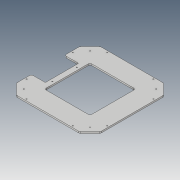
# Autodesk Inventor part: topPlate
Saved by Autodesk Inventor 2018 (Build 220112000, 112)
## iProperties
Created: 2019-11-22
Part Number: topPlate
Material: Generic
Document SubType Name: Modeling
Designer: anirudh
Density: 1 g/cm^3
Appearance: Default
Author: anirudh
Autodesk Inventor part; units mm, degrees
ref_plane "YZ Plane" through (0, 0, 0) normal (1, 0, 0) x (0, 1, 0)
ref_plane "XZ Plane" through (0, 0, 0) normal (0, 1, 0) x (-1, 0, 0)
ref_plane "XY Plane" through (0, 0, 0) normal (0, 0, 1) x (1, 0, 0)
sketch "Sketch1" plane through (0, 0, 0) normal (0, 1, 0) x (-1, 0, 0)
  line L0 (304.8, -38.1) -> (304.8, -266.7)
  line L1 (266.7, -304.8) -> (38.1, -304.8)
  line L2 (0, -266.7) -> (0, -38.1)
  line L3 (0, -38.1) -> (38.1, 0)
  line L4 (38.1, 0) -> (266.7, 0)
  line L5 (266.7, 0) -> (304.8, -38.1)
  line L6 (0, -266.7) -> (38.1, -304.8)
  line L7 (266.7, -304.8) -> (304.8, -266.7)
  circle A0 centre (238.125, -87.3125) radius 1.85
  circle A1 centre (66.675, -87.3125) radius 1.85
  circle A2 centre (66.675, -217.4875) radius 1.85
  circle A3 centre (238.125, -217.4875) radius 1.85
  point P0 (0, 0)
  dimension "d10" = 3.7
  dimension "d11" = 3.7
  dimension "d12" = 3.7
  dimension "d13" = 3.7
  constraints: 16 end point, 4 centre point, 1 parallel, 1 perpendicular
  measures "d10" diameter of A0
  measures "d11" diameter of A1
  measures "d12" diameter of A2
  measures "d13" diameter of A3
extrude "Extrusion1" add sketch "Sketch1" along normal blind 5.588
sketch "Sketch2" plane through (0, 5.588, 0) normal (0, 1, 0) x (1, 0, 0)
  line L0 (-304.8, 266.7) -> (-304.8, 38.1) projected
  line L1 (0, 38.1) -> (0, 266.7) projected
  line L2 (-152.4, 69.85) -> (-234.95, 69.85)
  line L3 (-234.95, 69.85) -> (-234.95, 234.95)
  line L4 (-234.95, 234.95) -> (-69.85, 234.95)
  line L5 (-69.85, 234.95) -> (-69.85, 69.85)
  line L6 (-69.85, 69.85) -> (-152.4, 69.85)
  point P0 (0, 0)
  dimension "d17" = 82.55
  dimension "d18" = 165.1
  dimension "d19" = 165.1
  dimension "d20" = 165.1
  constraints: 10 end point, 2 perpendicular, 1 collinear, 1 point on line
  measures "d17" distance of L2.start L2.end
  measures "d18" distance of L2.end L3.end
  measures "d19" distance of L3.end L4.end
  measures "d20" distance of L4.end L5.end
extrude "Extrusion2" cut sketch "Sketch2" against normal blind 25.4
sketch "Sketch3" plane through (0, 5.588, 0) normal (0, 1, 0) x (1, 0, 0)
  circle A0 centre (-238.125, 217.4875) radius 1.85 projected
  circle A1 centre (-238.125, 217.4875) radius 1.85
  circle A2 centre (-238.125, 87.3125) radius 1.85 projected
  circle A3 centre (-238.125, 87.3125) radius 1.85
  circle A4 centre (-66.675, 87.3125) radius 1.85 projected
  circle A5 centre (-66.675, 87.3125) radius 1.85
  circle A6 centre (-66.675, 217.4875) radius 1.85 projected
  circle A7 centre (-66.675, 217.4875) radius 1.85
  point P0 (0, 0)
  constraints: 4 centre point, 4 coincident
extrude "Extrusion3" add sketch "Sketch3" against normal blind 5.588
fillet "Fillet1" radius 6.35 4 edges at (-234.95, 2.794, -69.85) (-234.95, 2.794, -234.95) (-69.85, 2.794, -69.85) (-69.85, 2.794, -234.95)
fillet "Fillet2" radius 6.35 8 edges at (-38.1, 2.794, 0) (0, 2.794, -38.1) (0, 2.794, -266.7) (-38.1, 2.794, -304.8) (-266.7, 2.794, 0) (-304.8, 2.794, -38.1) (-304.8, 2.794, -266.7) (-266.7, 2.794, -304.8)
sketch "Sketch4" plane through (0, 5.588, 0) normal (0, 1, 0) x (1, 0, 0)
  circle A0 centre (-68.5771, 6.3529) radius 1.85
  circle A1 centre (-68.5771, 6.3529) radius 1.85
  circle A2 centre (-32.5204, 32.5204) radius 1.85
  circle A3 centre (-32.5204, 32.5204) radius 1.85
  circle A4 centre (-6.3529, 68.5771) radius 1.85
  circle A5 centre (-6.3529, 68.5771) radius 1.85
  line L0 (-304.8, 40.7303) -> (-304.8, 264.0697) projected
  line L1 (0, 264.0697) -> (0, 40.7303) projected
  line L2 (-40.7303, 304.8) -> (-264.0697, 304.8) projected
  line L3 (-40.7303, 0) -> (-264.0697, 0) projected
  circle A6 centre (-68.5771, 298.4471) radius 1.85
  circle A7 centre (-68.5771, 298.4471) radius 1.85
  circle A8 centre (-32.5204, 272.2796) radius 1.85
  circle A9 centre (-32.5204, 272.2796) radius 1.85
  circle A10 centre (-6.3529, 236.2229) radius 1.85
  circle A11 centre (-6.3529, 236.2229) radius 1.85
  circle A12 centre (-236.2229, 6.3529) radius 1.85
  circle A13 centre (-236.2229, 6.3529) radius 1.85
  circle A14 centre (-272.2796, 32.5204) radius 1.85
  circle A15 centre (-272.2796, 32.5204) radius 1.85
  circle A16 centre (-298.4471, 68.5771) radius 1.85
  circle A17 centre (-298.4471, 68.5771) radius 1.85
  circle A18 centre (-236.2229, 298.4471) radius 1.85
  circle A19 centre (-236.2229, 298.4471) radius 1.85
  circle A20 centre (-272.2796, 272.2796) radius 1.85
  circle A21 centre (-272.2796, 272.2796) radius 1.85
  circle A22 centre (-298.4471, 236.2229) radius 1.85
  circle A23 centre (-298.4471, 236.2229) radius 1.85
  point P0 (0, 0)
  point P1 (-1.8599, 36.2401)
  point P2 (-36.2401, 1.8599)
  point P3 (-47.0774, 8.9831)
  constraints: 24 centre point, 12 coincident
extrude "Extrusion4" cut sketch "Sketch4" against normal blind 13.5255
sketch "Sketch6" plane through (0, 5.588, 0) normal (0, 1, 0) x (1, 0, 0)
  line L0 (-304.8, 152.4) -> (-304.8, 212.725)
  line L1 (-304.8, 212.725) -> (-254, 212.725)
  line L2 (-254, 212.725) -> (-254, 92.075)
  line L3 (-254, 92.075) -> (-304.8, 92.075)
  line L4 (-304.8, 152.4) -> (-304.8, 92.075)
  line L5 (-304.8, 264.0697) -> (-304.8, 40.7303) projected
  point P0 (0, 0)
  dimension "d29" = 60.325
  dimension "d32" = 120.65
  constraints: 10 end point, 2 perpendicular, 1 collinear
  measures "d29" distance of L0.start L0.end
  measures "d32" distance of L1.end L2.end
extrude "Extrusion5" cut sketch "Sketch6" against normal blind 13.5255
fillet "Fillet4" radius 6.35 2 edges at (-304.8, 2.794, -92.075) (-304.8, 2.794, -212.725)
fillet "Fillet5" radius 3.175 2 edges at (-254, 2.794, -212.725) (-254, 2.794, -92.075)
sketch "Sketch7" plane through (0, 5.588, 0) normal (0, 1, 0) x (1, 0, 0)
  circle A0 centre (-244.475, 196.85) radius 1.85
  line L0 (-234.95, 76.2) -> (-234.95, 228.6) projected
  line L1 (-254, 95.25) -> (-254, 209.55) projected
  circle A1 centre (-244.475, 107.95) radius 1.85
  point P0 (0, 0)
  dimension "d53" = 3.7
  dimension "d59" = 3.7
  constraints: 2 centre point
  measures "d53" diameter of A0
  measures "d59" diameter of A1
extrude "Extrusion7" cut sketch "Sketch7" against normal blind 13.5255
body "Solid1"
